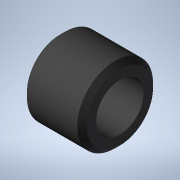
# Autodesk Inventor part: CLBPS5-8-6.3
Saved by Autodesk Inventor 2021 (Build 250183000, 183)
## iProperties
Created: 2025-06-12
Part Number: CLBPS5-8-6.3
Material: Generic
Catalog Web Link: www.cadenas.de
Description: CLBU, CLBUB, CLBUM, CLBUS,  CLBP, CLBPB, CLBPM, CLBPS-Bearing Spacers - For Inner Ring
Vendor: MISUMI
Document SubType Name: Modeling
Designer: psAdmin
Manufacturer: MISUMI
Mass: 0.186951 g
Surface Area: 3.03184 cm^2
Volume: 0.186951 cm^3
Density: 1 g/cm^3
Appearance: PSOLRGB-191-191-191
Category: PARTsolutions
Company: MISUMI
Title: CLBPS5-8-6.3
Author: Cadenas PARTsolutions
Comments: Bearing Spacers - For Inner Ring
PSOL_IDENT_0: {$CADENAS_DATA/23d-libs/misumi/metric/12_bearing_holders/clbu.prj},236 {VTYP=3D},{NB=CLBPS5-8-6.3},{
PSOL_IDENT_1: LINA=CLBPS5-8-6.3},{NN=CLBU, CLBUB, CLBUM, CLBUS,  CLBP, CLBPB, CLBPM, CLBPS},{DATE=09.09.2019 15:26
PSOL_IDENT_2: :56},{GEOMDATE=08.10.2015 00:14:34},{VERSION=},{LINEID=30},{WBVAR=LTOL,MAT,ST,DD,L,ALT1},{WBNUMERIC=
PSOL_IDENT_3: DD,L}  {NB=CLBPS5-8-6.3},{LINA=CLBPS5-8-6.3},{KT=DUMMY},{PN=CLBPS5-8-6.3},{TYPE=CLBPS},{TS11=3},{LTO
PSOL_IDENT_4: L=P},{MAT=S},{MATALG= '', 'Aluminum Alloy 5000 series', 'BM', 'Low Carbon Steel', 'S' , 'SUS304' },{
PSOL_IDENT_5: ST=},{ST1=   '','-'         },{D=8},{D1=8},{DD=5},{L=6.3},{L1= [1.0:50.0/0.1]},{ALT1=},{ALT1ALG='','
PSOL_IDENT_6: w/o UKC (Overall Length Tolerance)','-UKC','with UKC (Overall Length Tolerance)'},{LTOL1=+0.1/0},{DS
PSOL_IDENT_7: S=7},{DD1=5},{AP=695ZZ,605ZZ,625ZZ,675ZZ},{LTEMP=},{DPN=8},{DSSPN=CLBPS58-6.3},{ALT1PN=},{DDPN=5},{C
PSOL_IDENT_8: OLOR=0.75,0.75,0.75,0.00}
NB: CLBPS5-8-6.3
NN: CLBU, CLBUB, CLBUM, CLBUS,  CLBP, CLBPB, CLBPM, CLBPS
NT: Bearing Spacers - For Inner Ring
NBSYN: $PN.
LINA: CLBPS5-8-6.3
CATALOG: Misumi
PN: CLBPS5-8-6.3
LTOL: Plus Tolerance
MAT: SUS304
ST: -
D: 8
DD: 5
L: 6.3
ALT1: w/o UKC (Overall Length Tolerance)
DSS: 7
AP: 695ZZ,605ZZ,625ZZ,675ZZ
SUPPLIER: MISUMI
ARTICLENO: CLBPS5-8-6.3
BOMINFO: CLBPS5-8-6.3
CREATOR: CADENAS GmbH
Autodesk Inventor part; units mm, degrees
sketch "Sketch_1" plane through (0, 0, 0) normal (0, 0, 1) x (1, 0, 0)
  line L0 (6.3, 0) -> (0, 0)
  line L1 (0, 2.5) -> (6.3, 2.5)
  line L2 (6.3, 2.5) -> (6.3, 3.5)
  line L3 (6.3, 3.5) -> (5.8, 4)
  line L4 (5.8, 4) -> (0.5, 4)
  line L5 (0.5, 4) -> (0, 3.5)
  line L6 (0, 3.5) -> (0, 2.5)
  constraints: 14 end point
revolve "Revolution1" add sketch "Sketch_1" angle 360 about axis through (6.3, 0, 0) along (1, 0, 0)
ref_plane "to_b_XY" through (0, 0, 0) normal (1, 0, 0) x (0, 0, -1)
ref_plane "to_b_YZ" through (0, 0, 0) normal (0, 0, -1) x (0, 1, 0)
ref_plane "to_b_ZX" through (0, 0, 0) normal (0, 1, 0) x (1, 0, 0)
body "Solid1"
